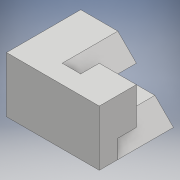
# Autodesk Inventor part: 17
Saved by Autodesk Inventor 2017 (Build 210142000, 142)
## iProperties
Part Number: 17
Material: 一般
Document SubType Name: Modeling
Designer: Brian
Density: 1 g/cm^3
Appearance: 預設
Author: Brian
Autodesk Inventor part; units mm, degrees
ref_plane "YZ Plane" through (0, 0, 0) normal (1, 0, 0) x (0, 1, 0)
ref_plane "XZ Plane" through (0, 0, 0) normal (0, 1, 0) x (-1, 0, 0)
ref_plane "XY Plane" through (0, 0, 0) normal (0, 0, 1) x (1, 0, 0)
sketch "草圖1" plane through (0, 0, 0) normal (0, 1, 0) x (-1, 0, 0)
  line L0 (0, 0) -> (-50, 0)
  line L1 (-50, 0) -> (-50, -30)
  line L2 (-50, -30) -> (0, -30)
  line L3 (0, -30) -> (0, 0)
  dimension "d0" = 30
  dimension "d1" = 50
  constraints: 8 end point, 2 parallel, 1 horizontal, 1 perpendicular
  measures "d0" distance of L2.end L0.start
  measures "d1" distance of L1.end L2.end
extrude "擠出1" add sketch "草圖1" along normal blind 40
sketch "草圖2" plane through (50, 0, 0) normal (1, 0, 0) x (0, 0, -1)
  line L0 (0, 40) -> (30, 40) projected
  line L1 (10, 40) -> (20, 40)
  line L2 (20, 40) -> (20, 30)
  line L3 (20, 30) -> (10, 30)
  line L4 (10, 30) -> (10, 40)
  point P0 (0, 0)
  dimension "d4" = 10
  dimension "d5" = 10
  dimension "d6" = 10
  constraints: 8 end point, 2 parallel, 1 horizontal, 1 perpendicular, 1 point on line
  measures "d4" distance of L2.end L3.end
  measures "d5" distance of L3.end L1.start
  measures "d6" distance from line of L0.start L4
extrude "擠出2" cut sketch "草圖2" against normal through all
sketch "草圖3" plane through (0, 40, 0) normal (0, 1, 0) x (1, 0, 0)
  line L0 (50, 0) -> (50, 30) projected
  line L1 (50, 30) -> (20, 0)
  line L2 (0, 0) -> (50, 0) projected
  line L3 (50, 20) -> (30, 0)
  line L4 (20, 0) -> (30, 0)
  line L5 (50, 30) -> (50, 20)
  dimension "d9" = 10
  dimension "d10" = 135
  constraints: 8 end point, 5 point on line, 1 parallel, 1 vertical
  measures "d9" distance of L1.end L3.end
  measures "d10" angle of L2 L1
extrude "擠出3" cut sketch "草圖3" against normal blind 30 contours L3 L2 L1 L0
sketch "草圖4" plane through (0, 40, 0) normal (0, 1, 0) x (1, 0, 0)
  line L0 (40, 10) -> (30, 0) projected
  line L1 (30, 0) -> (50, 0) projected
  line L2 (50, 0) -> (50, 10) projected
  line L3 (50, 10) -> (40, 10) projected
  line L4 (50, 20) -> (40, 10) projected
  line L5 (50, 10) -> (40, 10) projected
  line L6 (50, 20) -> (50, 10) projected
  point P0 (0, 0)
extrude "擠出4" cut sketch "草圖4" against normal blind 20
